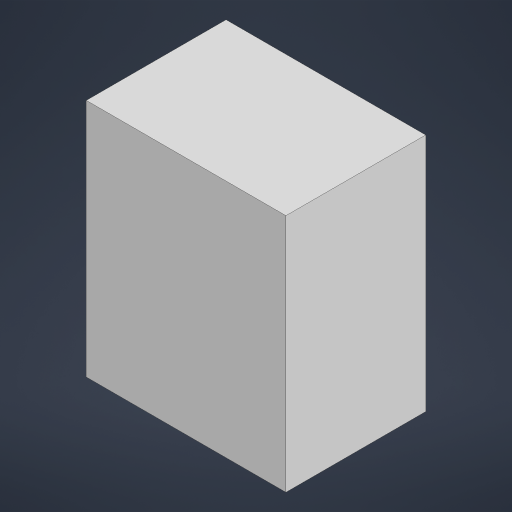
# Autodesk Inventor part: Compressor
Saved by Autodesk Inventor 2023 (Build 270158000, 158)
## iProperties
Created: 2023-09-15
Part Number: Compressor
Material: Generic
Document SubType Name: Modeling
Designer: Abhinav
Density: 1 g/cm^3
Appearance: Default
Author: Abhinav
Autodesk Inventor part; units mm, degrees
ref_plane "YZ Plane" through (0, 0, 0) normal (1, 0, 0) x (0, 1, 0)
ref_plane "XZ Plane" through (0, 0, 0) normal (0, 1, 0) x (-1, 0, 0)
ref_plane "XY Plane" through (0, 0, 0) normal (0, 0, 1) x (1, 0, 0)
sketch "Sketch1" plane through (0, 0, 0) normal (0, 1, 0) x (-1, 0, 0)
  line L0 (25, 17.5) -> (-25, 17.5)
  line L1 (-25, 17.5) -> (-25, -17.5)
  line L2 (-25, -17.5) -> (25, -17.5)
  line L3 (25, -17.5) -> (25, 17.5)
  line L4 (25, 17.5) -> (-25, -17.5) construction
  line L5 (-25, 17.5) -> (25, -17.5) construction
  point P0 (0, 0)
  dimension "d0" = 50
  dimension "d1" = 35
  constraints: 12 end point, 2 midpoint, 2 parallel, 1 horizontal, 1 perpendicular
  measures "d0" distance of L2.end L1.end
  measures "d1" distance of L1.end L0.end
extrude "Extrusion1" add sketch "Sketch1" along normal blind 60
body "Solid1"
